Autodesk Inventor part; units mm, degrees
(part 2 of 2)
extrude "押し出し11" add sketch "スケッチ9" against normal up to surface (7.6939 mm away) contours L2 L13 L6 L0
sketch "スケッチ13" plane through (0, 0, 1.5) normal (0, 0, 1) x (1, 0, 0)
  line L0 (-15.3278, 9.5528) -> (-16.1644, 1.5927) projected
  line L1 (-16.1644, 1.5927) -> (-17.5005, 9.1697) projected
  line L2 (-15.3278, 9.5528) -> (-17.5005, 9.1697) projected
  point P0 (0, 0)
extrude "押し出し12" cut sketch "スケッチ13" along normal blind 8
mirror "ミラー1" about plane through (0, 0, 0) normal (1, 0, 0) of "押し出し12", "押し出し11"
chamfer "面取り4" distance 0.8 angle 45 2 edges at (-2.1443, 9.6497, 1.5) (2.1443, 9.6497, 1.5)
chamfer "面取り5" distance 0.8 angle 45 2 edges at (1.5375, 10.449, 0.7818) (-1.5375, 10.449, 0.7818)
chamfer "面取り6" distance 1 angle 45 2 edges at (7.7859, 4.2124, 7) (-7.7859, 4.2124, 7)
extrude "押し出し13" cut sketch "スケッチ6" along normal blind 0.4 contours A6 L0 | L0 A6 | A7 L10 | L10 A7
extrude "押し出し14" add sketch "スケッチ6" along normal up to surface (1.5 mm away) contours A2
extrude "押し出し15" add sketch "スケッチ6" along normal up to surface (1.5 mm away) contours A4
extrude "押し出し16" add sketch "スケッチ6" along normal up to surface (1.5 mm away) contours A1
chamfer "面取り7" distance 0.8 angle 45 2 edges at (-14.7312, 1.8454, 1.5) (14.7312, 1.8454, 1.5)
extrude "押し出し17" cut sketch "スケッチ8" against normal blind 10 contours A1
extrude "押し出し18" cut sketch "スケッチ7" against normal blind 10 contours A1
extrude "押し出し19" cut sketch "スケッチ8" against normal blind 10 contours L12 L1 L18 L0 | L0 L18 L12 | L12 L2 L18 L1
extrude "押し出し20" cut sketch "スケッチ7" against normal blind 10 contours L7 L2 L4 L19 | L4 L2 L5 L19 | L5 L2 L19
ref_plane "作業平面5" through (0, 0, 1.5) normal (0, 0, -1) x (-1, 0, 0)
ref_plane "作業平面6" through (7.5905, 3.1045, 0) normal (0.1736482, 0.9848078, 0) x (-0.9848078, 0.1736482, 0)
equation "\"d42\" = d41"
